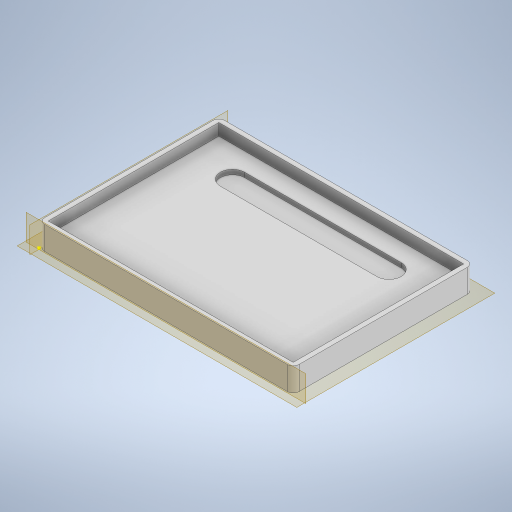
# Autodesk Inventor part: mag_case_v3
Saved by Autodesk Inventor 2024 (Build 280153000, 153)
## iProperties
Created: 2023-11-21
Part Number: mag_case_v3
Material: Generic
Document SubType Name: Modeling
Designer: sophi
Density: 1 g/cm^3
Appearance: Default
Author: sophi
Autodesk Inventor part; units mm, degrees
sketch "Sketch1" plane through (0, 0, 0) normal (0, 1, 0) x (-1, 0, 0)
  point P0 (0, 0)
sketch "Sketch2" plane through (0, 0, 0) normal (0, 1, 0) x (-1, 0, 0)
  line L0 (0, 0) -> (-65, 0)
  line L1 (-65, 0) -> (-65, -46)
  line L2 (-65, -46) -> (0, -46)
  line L3 (0, -46) -> (0, 0)
  dimension "d0" = 65
  dimension "d1" = 46
  constraints: 8 end point, 2 parallel, 1 horizontal, 1 perpendicular
  measures "d0" distance of L1.end L2.end
  measures "d1" distance of L0.end L1.end
extrude "Extrusion1" add sketch "Sketch2" along normal blind 3
sketch "Sketch3" plane through (0, 3, 0) normal (0, 1, 0) x (1, 0, 0)
  circle A0 centre (32.5, 37) radius 3.1
  line L0 (65, 46) -> (0, 46) projected
  line L1 (65, 0) -> (65, 46) projected
  line L2 (12.5, 40.1) -> (52.5, 40.1)
  line L3 (0, 46) -> (0, 0) projected
  line L4 (12.5, 33.9) -> (52.5, 33.9)
  arc A1 (12.5, 40.1) -> (12.5, 33.9) centre (12.5, 37) ccw
  arc A2 (52.5, 33.9) -> (52.5, 40.1) centre (52.5, 37) ccw
  point P0 (63.5, 46)
  point P1 (1.5, 46)
  point P2 (32.5, 46)
  point P3 (32.5, 46)
  point P4 (32.5, 46)
  point P5 (32.5, 40.1)
  point P6 (32.5, 40.1)
  point P7 (32.5, 33.9)
  dimension "d5" = 6.2
  dimension "d6" = 0
  dimension "d7" = 9
  dimension "d18" = 40
  dimension "d19" = 0
  constraints: 6 tangent, 4 end point, 4 midpoint, 4 point on circle, 3 centre point, 2 horizontal
  measures "d5" diameter of A0
  measures "d6" horizontal distance of point (32.5, 46) A0.centre
  measures "d7" distance of point (32.5, 46) A0.centre
  measures "d18" distance of L2.start L2.end
  measures "d19" horizontal distance of point (32.5, 46) point (32.5, 40.1)
extrude "Extrusion2" cut sketch "Sketch3" against normal blind 1.2
sketch "Sketch6" plane through (0, 3, 0) normal (0, 1, 0) x (1, 0, 0)
  line L0 (0, 0) -> (65, 0) projected
  line L1 (65, 0) -> (65, 46) projected
  line L2 (0, 0) -> (65, 0)
  line L3 (65, 0) -> (65, 46)
  line L4 (65, 46) -> (0, 46)
  line L5 (0, 46) -> (0, 0)
  line L6 (1.2, 44.8) -> (63.8, 44.8)
  line L7 (63.8, 44.8) -> (63.8, 1.2)
  line L8 (63.8, 1.2) -> (1.2, 1.2)
  line L9 (1.2, 1.2) -> (1.2, 44.8)
  dimension "d13" = 1.2
  constraints: 16 end point, 4 parallel, 2 perpendicular, 1 horizontal, 3 other
  measures "d13" distance between parallel lines of L4 L6
extrude "Extrusion4" add sketch "Sketch6" along normal blind 3
fillet "Fillet2" radius 1.5 4 edges at (0, 3, 0) (65, 3, 0) (65, 3, -46) (0, 3, -46)
equation "\"d0\" = length + thickness"
equation "\"d1\" = width + thickness"
equation "\"d2\" = thickness"
equation "\"d5\" = mag_diameter"
equation "\"d8\" = mag_thickness"
equation "\"d13\" = 0.4 * thickness"
equation "\"d14\" = thickness"
equation "\"d16\" = 0.5 * thickness"
equation "\"length\" = 62"
equation "\"width\" = 43"
equation "\"thickness\" = 3"
equation "\"mag_thickness\" = 1.2"
equation "\"mag_diameter\" = 6.2"
body "Solid1"
